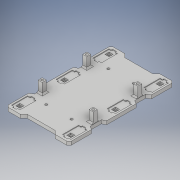
# Autodesk Inventor part: BODY_BOTTOM
Saved by Autodesk Inventor 2017.3 (Build 213256000, 256)
## iProperties
Created: 2017-08-24
Part Number: BODY_BOTTOM
Material: Generic
Document SubType Name: Modeling
Designer: Alexander Miller
Density: 1 g/cm^3
Appearance: Default
body_A: 150,000 mm
body_B: 90,000 mm
body_C: 5,000 mm
Author: Alexander Miller
Autodesk Inventor part; units mm, degrees
ref_plane "YZ Plane" through (0, 0, 0) normal (1, 0, 0) x (0, 1, 0)
ref_plane "XZ Plane" through (0, 0, 0) normal (0, 1, 0) x (-1, 0, 0)
ref_plane "XY Plane" through (0, 0, 0) normal (0, 0, 1) x (1, 0, 0)
sketch "Sketch4" plane through (0, 0, 0) normal (0, 1, 0) x (-1, 0, 0)
  line L0 (45, 75) -> (-45, 75)
  line L1 (-45, 75) -> (-45, -75)
  line L2 (-45, -75) -> (45, -75)
  line L3 (45, -75) -> (45, 75)
  point P0 (0, 0)
  point P1 (0, -75)
  point P2 (45, 0)
  dimension "d15" = 150
  dimension "d16" = 90
  constraints: 8 end point, 2 midpoint, 2 parallel, 1 horizontal, 1 horizontal alignment, 1 perpendicular, 1 vertical alignment
  measures "d15" distance of L2.end L0.start
  measures "d16" distance of L1.end L2.end
extrude "BodyPlate" add sketch "Sketch4" along normal blind 5
sketch "Sketch5" plane through (0, 5, 0) normal (0, 1, 0) x (1, 0, 0)
  line L0 (-42.5, 69.75) -> (-30.5, 69.75)
  line L1 (-30.5, 69.75) -> (-30.5, 46.75)
  line L2 (-30.5, 46.75) -> (-42.5, 46.75)
  line L3 (-42.5, 46.75) -> (-42.5, 69.75)
  line L4 (-42.5, 17) -> (-30.5, 17)
  line L5 (-30.5, 17) -> (-30.5, -6)
  line L6 (-30.5, -6) -> (-42.5, -6)
  line L7 (-42.5, -6) -> (-42.5, 17)
  line L8 (-42.5, -46.75) -> (-30.5, -46.75)
  line L9 (-30.5, -46.75) -> (-30.5, -69.75)
  line L10 (-30.5, -69.75) -> (-42.5, -69.75)
  line L11 (-42.5, -69.75) -> (-42.5, -46.75)
  line L12 (45, 75) -> (-45, 75) projected
  line L13 (-45, 75) -> (-45, -75) projected
  line L14 (-45, -75) -> (45, -75) projected
  circle A0 centre (-36.5, 0) radius 6 construction
  line L15 (0, 105) -> (0, -105) construction
  line L16 (42.5, 69.75) -> (30.5, 69.75)
  line L17 (30.5, 69.75) -> (30.5, 46.75)
  line L18 (30.5, 46.75) -> (42.5, 46.75)
  line L19 (42.5, 46.75) -> (42.5, 69.75)
  line L20 (42.5, 17) -> (30.5, 17)
  line L21 (30.5, 17) -> (30.5, -6)
  line L22 (30.5, -6) -> (42.5, -6)
  line L23 (42.5, -6) -> (42.5, 17)
  line L24 (42.5, -46.75) -> (30.5, -46.75)
  line L25 (30.5, -46.75) -> (30.5, -69.75)
  line L26 (30.5, -69.75) -> (42.5, -69.75)
  line L27 (42.5, -69.75) -> (42.5, -46.75)
  point P0 (0, 0)
  point P1 (-36.5, 46.75)
  point P2 (-36.5, 17)
  point P3 (-36.5, -6)
  point P4 (-36.5, -46.75)
  dimension "d19" = 23
  dimension "d20" = 12
  dimension "d21" = 5.25
  dimension "d22" = 2.5
  dimension "d23" = 5.25
  constraints: 48 end point, 12 symmetric about line, 6 parallel, 4 equal length, 4 midpoint, 3 horizontal, 3 perpendicular, 3 tangent, 2 vertical alignment, 1 centre point, 1 horizontal alignment
  measures "d19" distance of L2.end L0.start
  measures "d20" distance of L0.start L0.end
  measures "d21" distance between parallel lines of L0 L12
  measures "d22" distance between parallel lines of L3 L13
  measures "d23" distance between parallel lines of L14 L10
extrude "ServoIndentation" cut sketch "Sketch5" against normal blind 1
sketch "Sketch6" plane through (0, 5, 0) normal (0, 1, 0) x (1, 0, 0)
  line L0 (-39, 71.75) -> (-34, 71.75)
  line L1 (-34, 71.75) -> (-34, 69.75)
  line L2 (-34, 69.75) -> (-39, 69.75)
  line L3 (-39, 69.75) -> (-39, 71.75)
  line L4 (-39, 46.75) -> (-34, 46.75)
  line L5 (-34, 46.75) -> (-34, 44.75)
  line L6 (-34, 44.75) -> (-39, 44.75)
  line L7 (-39, 44.75) -> (-39, 46.75)
  line L8 (-42.5, 69.75) -> (-30.5, 69.75) projected
  line L9 (-30.5, 46.75) -> (-42.5, 46.75) projected
  line L10 (-39, 19) -> (-34, 19)
  line L11 (-34, 19) -> (-34, 17)
  line L12 (-34, 17) -> (-39, 17)
  line L13 (-39, 17) -> (-39, 19)
  line L14 (-39, -6) -> (-34, -6)
  line L15 (-34, -6) -> (-34, -8)
  line L16 (-34, -8) -> (-39, -8)
  line L17 (-39, -8) -> (-39, -6)
  line L18 (-39, -44.75) -> (-34, -44.75)
  line L19 (-34, -44.75) -> (-34, -46.75)
  line L20 (-34, -46.75) -> (-39, -46.75)
  line L21 (-39, -46.75) -> (-39, -44.75)
  line L22 (-39, -69.75) -> (-34, -69.75)
  line L23 (-34, -69.75) -> (-34, -71.75)
  line L24 (-34, -71.75) -> (-39, -71.75)
  line L25 (-39, -71.75) -> (-39, -69.75)
  line L26 (-42.5, 17) -> (-30.5, 17) projected
  line L27 (-30.5, -6) -> (-42.5, -6) projected
  line L28 (-42.5, -46.75) -> (-30.5, -46.75) projected
  line L29 (-30.5, -69.75) -> (-42.5, -69.75) projected
  line L30 (0, 105) -> (0, -105) projected
  line L31 (39, 71.75) -> (34, 71.75)
  line L32 (34, 71.75) -> (34, 69.75)
  line L33 (34, 69.75) -> (39, 69.75)
  line L34 (39, 69.75) -> (39, 71.75)
  line L35 (39, 46.75) -> (34, 46.75)
  line L36 (34, 46.75) -> (34, 44.75)
  line L37 (34, 44.75) -> (39, 44.75)
  line L38 (39, 44.75) -> (39, 46.75)
  line L39 (39, 19) -> (34, 19)
  line L40 (34, 19) -> (34, 17)
  line L41 (34, 17) -> (39, 17)
  line L42 (39, 17) -> (39, 19)
  line L43 (39, -6) -> (34, -6)
  line L44 (34, -6) -> (34, -8)
  line L45 (34, -8) -> (39, -8)
  line L46 (39, -8) -> (39, -6)
  line L47 (39, -44.75) -> (34, -44.75)
  line L48 (34, -44.75) -> (34, -46.75)
  line L49 (34, -46.75) -> (39, -46.75)
  line L50 (39, -46.75) -> (39, -44.75)
  line L51 (39, -69.75) -> (34, -69.75)
  line L52 (34, -69.75) -> (34, -71.75)
  line L53 (34, -71.75) -> (39, -71.75)
  line L54 (39, -71.75) -> (39, -69.75)
  point P0 (0, 0)
  point P1 (-36.5, 69.75)
  point P2 (-36.5, 69.75)
  point P3 (-36.5, 46.75)
  point P4 (-36.5, 46.75)
  point P5 (-36.5, 17)
  point P6 (-36.5, 17)
  point P7 (-36.5, -6)
  point P8 (-36.5, -6)
  point P9 (-36.5, -46.75)
  point P10 (-36.5, -46.75)
  point P11 (-36.5, -69.75)
  point P12 (-36.5, -69.75)
  dimension "d28" = 2
  dimension "d29" = 5
  constraints: 96 end point, 24 symmetric about line, 12 midpoint, 12 parallel, 9 equal length, 6 coincident, 6 collinear, 6 horizontal, 6 perpendicular, 2 point on line
  measures "d28" distance of L2.end L0.start
  measures "d29" distance of L0.start L0.end
extrude "ServoCableIdentation" cut sketch "Sketch6" against normal up to surface (1 mm away)
fillet "ServoCableFillet" radius 0.75 24 edges at (-39, 4.5, -69.75) (-34, 4.5, -69.75) (-39, 4.5, -46.75) (-34, 4.5, -46.75) (-39, 4.5, -17) (-34, 4.5, -17) (-39, 4.5, 6) (-34, 4.5, 6) (-39, 4.5, 46.75) (-34, 4.5, 46.75) (-39, 4.5, 69.75) (-34, 4.5, 69.75) (34, 4.5, -69.75) (39, 4.5, -69.75) (34, 4.5, -46.75) (39, 4.5, -46.75) (34, 4.5, -17) (39, 4.5, -17) (34, 4.5, 6) (39, 4.5, 6) (34, 4.5, 46.75) (39, 4.5, 46.75) (34, 4.5, 69.75) (39, 4.5, 69.75)
sketch "Sketch7" plane through (0, 5, 0) normal (0, 1, 0) x (1, 0, 0)
  line L0 (45, 75) -> (-45, 75) projected
  circle A0 centre (-18.1, 44.45) radius 1.675
  circle A1 centre (-18.1, -44.45) radius 1.675
  circle A2 centre (18.1, 44.45) radius 1.675
  circle A3 centre (18.1, -44.45) radius 1.675
  line L1 (-18.1, -44.45) -> (18.1, -44.45) construction
  line L2 (18.1, -44.45) -> (18.1, 44.45) construction
  line L3 (18.1, 44.45) -> (-18.1, 44.45) construction
  line L4 (-18.1, 44.45) -> (-18.1, -44.45) construction
  point P0 (0, 0)
  point P1 (-18.1, 0)
  point P2 (0, 44.45)
  dimension "d40" = 88.9
  dimension "d63" = 36.2
  dimension "d65" = 3.35
  constraints: 8 end point, 4 centre point, 3 equal radius, 3 horizontal alignment, 3 vertical alignment, 2 midpoint, 2 parallel, 1 horizontal, 1 perpendicular
  measures "d40" distance of A0.centre L1.start
  measures "d63" distance of A3.centre L1.start
  measures "d65" diameter of A0
extrude "PCBMounting" cut sketch "Sketch7" against normal through all
sketch "Sketch8" plane through (0, 0, 0) normal (0, -1, 0) x (1, 0, 0)
  circle A0 centre (18.1, -44.45) radius 1.675 projected
  circle A1 centre (-18.1, -44.45) radius 1.675 projected
  circle A2 centre (-18.1, 44.45) radius 1.675 projected
  circle A3 centre (18.1, 44.45) radius 1.675 projected
  line L0 (15.175, 47.375) -> (21.025, 47.375)
  line L1 (21.025, 47.375) -> (21.025, 41.525)
  line L2 (21.025, 41.525) -> (15.175, 41.525)
  line L3 (15.175, 41.525) -> (15.175, 47.375)
  line L4 (15.175, -41.525) -> (21.025, -41.525)
  line L5 (21.025, -41.525) -> (21.025, -47.375)
  line L6 (21.025, -47.375) -> (15.175, -47.375)
  line L7 (15.175, -47.375) -> (15.175, -41.525)
  line L8 (-21.025, -41.525) -> (-15.175, -41.525)
  line L9 (-15.175, -41.525) -> (-15.175, -47.375)
  line L10 (-15.175, -47.375) -> (-21.025, -47.375)
  line L11 (-21.025, -47.375) -> (-21.025, -41.525)
  line L12 (-21.025, 47.375) -> (-15.175, 47.375)
  line L13 (-15.175, 47.375) -> (-15.175, 41.525)
  line L14 (-15.175, 41.525) -> (-21.025, 41.525)
  line L15 (-21.025, 41.525) -> (-21.025, 47.375)
  point P0 (0, 0)
  point P1 (15.175, 44.45)
  point P2 (-15.175, 44.45)
  point P3 (-15.175, -44.45)
  point P4 (15.175, -44.45)
  point P5 (18.1, 41.525)
  point P6 (18.1, -41.525)
  point P7 (-18.1, -41.525)
  point P8 (-18.1, 41.525)
  dimension "d64" = 5.85
  constraints: 32 end point, 8 midpoint, 8 parallel, 6 equal length, 4 horizontal, 4 horizontal alignment, 4 perpendicular, 4 vertical alignment, 1 point on line
  measures "d64" distance of L1.end L2.end
extrude "PCBNuts" cut sketch "Sketch8" against normal blind 2.15
sketch "Sketch9" plane through (0, 5, 0) normal (0, 1, 0) x (1, 0, 0)
  line L0 (45, 42.875) -> (45, 20.875)
  line L1 (45, 20.875) -> (40, 23.875)
  line L2 (40, 23.875) -> (40, 39.875)
  line L3 (40, 39.875) -> (45, 42.875)
  line L4 (34, 44.75) -> (39, 44.75) projected
  line L5 (36.5, 44.75) -> (36.5, 19) construction
  line L6 (39, 19) -> (34, 19) projected
  line L7 (45, -75) -> (45, 75) projected
  line L8 (-63, 0) -> (63, 0) projected
  line L9 (0, 105) -> (0, -105) projected
  line L10 (-45, 42.875) -> (-45, 20.875)
  line L11 (-45, 20.875) -> (-40, 23.875)
  line L12 (-40, 23.875) -> (-40, 39.875)
  line L13 (-40, 39.875) -> (-45, 42.875)
  line L14 (25, 75) -> (-25, 75)
  line L15 (-25, 75) -> (-20, 70)
  line L16 (-20, 70) -> (20, 70)
  line L17 (20, 70) -> (25, 75)
  line L18 (45, 75) -> (-45, 75) projected
  line L19 (45, -42.875) -> (45, -20.875)
  line L20 (45, -20.875) -> (40, -23.875)
  line L21 (40, -23.875) -> (40, -39.875)
  line L22 (40, -39.875) -> (45, -42.875)
  line L23 (-40, -39.875) -> (-45, -42.875)
  line L24 (-45, -42.875) -> (-45, -20.875)
  line L25 (-45, -20.875) -> (-40, -23.875)
  line L26 (-40, -23.875) -> (-40, -39.875)
  line L27 (25, -75) -> (-25, -75)
  line L28 (-25, -75) -> (-20, -70)
  line L29 (-20, -70) -> (20, -70)
  line L30 (20, -70) -> (25, -75)
  point P0 (0, 0)
  point P1 (45, 31.875)
  point P2 (40, 31.875)
  point P3 (36.5, 31.875)
  point P4 (0, 75)
  point P5 (0, 70)
  dimension "d46" = 5
  dimension "d47" = 16
  dimension "d48" = 22
  dimension "d49" = 5
  dimension "d50" = 40
  dimension "d51" = 50
  constraints: 50 end point, 16 symmetric about line, 7 midpoint, 2 collinear, 2 horizontal alignment, 2 parallel, 2 vertical alignment, 1 horizontal, 1 vertical
  measures "d46" distance between parallel lines of L2 L0
  measures "d47" distance of L1.end L2.end
  measures "d48" distance of L0.start L0.end
  measures "d49" distance between parallel lines of L16 L14
  measures "d50" distance of L15.end L16.end
  measures "d51" distance of L14.start L14.end
extrude "BodyIndentation" cut sketch "Sketch9" against normal through all contours L0 L1 L2 L3 | L17 L16 L9 L14 | L9 L16 L15 L14 | L22 L21 L20 L7 | L29 L30 L27 L9 | L9 L27 L28 L29 | L13 L12 L11 L10 | L23 L24 L25 L26
chamfer "BodyChamfer" distance 3 angle 45 4 edges at (-45, 2.5, 75) (-45, 2.5, -75) (45, 2.5, 75) (45, 2.5, -75)
sketch "Sketch10" plane through (0, 4, 0) normal (0, 1, 0) x (1, 0, 0)
  line L0 (-39.425, 66.675) -> (-33.575, 66.675)
  line L1 (-33.575, 66.675) -> (-33.575, 60.825)
  line L2 (-33.575, 60.825) -> (-39.425, 60.825)
  line L3 (-39.425, 60.825) -> (-39.425, 66.675)
  line L4 (-39.425, -2.925) -> (-33.575, -2.925)
  line L5 (-33.575, -2.925) -> (-33.575, 2.925)
  line L6 (-33.575, 2.925) -> (-39.425, 2.925)
  line L7 (-39.425, 2.925) -> (-39.425, -2.925)
  line L8 (-39.425, -66.675) -> (-33.575, -66.675)
  line L9 (-33.575, -66.675) -> (-33.575, -60.825)
  line L10 (-33.575, -60.825) -> (-39.425, -60.825)
  line L11 (-39.425, -60.825) -> (-39.425, -66.675)
  line L12 (-42.5, 46.75) -> (-42.5, 69.75) construction
  line L13 (-33.25, 69.75) -> (-30.5, 69.75) construction
  line L14 (-42.5, 69.75) -> (-30.5, 69.75) construction
  circle A0 centre (-36.5, 63.75) radius 6 construction
  line L15 (-30.5, 69.75) -> (-30.5, 46.75) construction
  line L16 (-39.75, -6) -> (-42.5, -6) construction
  line L17 (-42.5, -6) -> (-30.5, -6) construction
  circle A1 centre (-36.5, 0) radius 6 construction
  line L18 (-42.5, -6) -> (-42.5, 17) construction
  line L19 (-30.5, 17) -> (-30.5, -6) construction
  line L20 (-30.5, -46.75) -> (-30.5, -69.75) construction
  line L21 (-42.5, -69.75) -> (-42.5, -46.75) construction
  line L22 (-30.5, -69.75) -> (-42.5, -69.75) construction
  circle A2 centre (-36.5, -63.75) radius 6 construction
  line L23 (0, 105) -> (0, -105) construction
  line L24 (39.425, 66.675) -> (33.575, 66.675)
  line L25 (33.575, 66.675) -> (33.575, 60.825)
  line L26 (33.575, 60.825) -> (39.425, 60.825)
  line L27 (39.425, 60.825) -> (39.425, 66.675)
  line L28 (39.425, -2.925) -> (33.575, -2.925)
  line L29 (33.575, -2.925) -> (33.575, 2.925)
  line L30 (33.575, 2.925) -> (39.425, 2.925)
  line L31 (39.425, 2.925) -> (39.425, -2.925)
  line L32 (39.425, -66.675) -> (33.575, -66.675)
  line L33 (33.575, -66.675) -> (33.575, -60.825)
  line L34 (33.575, -60.825) -> (39.425, -60.825)
  line L35 (39.425, -60.825) -> (39.425, -66.675)
  point P0 (0, 0)
  point P1 (-36.5, 60.825)
  point P2 (-36.5, 2.925)
  point P3 (-36.5, -2.925)
  point P4 (-36.5, -60.825)
  point P5 (-36.5, 69.75)
  point P6 (-39.425, 63.75)
  point P7 (-36.5, 66.675)
  point P8 (-33.575, 0)
  point P9 (-33.575, -63.75)
  point P10 (36.5, 60.825)
  point P11 (36.5, 2.925)
  point P12 (36.5, -2.925)
  point P13 (36.5, -60.825)
  point P14 (36.5, 63.75)
  point P15 (39.425, 63.75)
  point P16 (36.5, 66.675)
  point P17 (36.5, 0)
  point P18 (33.575, 0)
  point P19 (36.5, -63.75)
  point P20 (33.575, -63.75)
  dimension "d57" = 5.85
  constraints: 54 end point, 23 symmetric about line, 9 midpoint, 8 perpendicular, 8 tangent, 6 parallel, 4 horizontal, 4 vertical alignment, 3 centre point, 3 horizontal alignment, 2 collinear
  measures "d57" distance of L0.end L1.end
extrude "BallbearingNut" cut sketch "Sketch10" against normal blind 2.15
sketch "Sketch11" plane through (0, 1.85, 0) normal (0, 1, 0) x (1, 0, 0)
  circle A0 centre (-36.5, -63.75) radius 1.675
  circle A1 centre (-36.5, 0) radius 1.675
  circle A2 centre (-36.5, 63.75) radius 1.675
  line L0 (0, 105) -> (0, -105) projected
  line L1 (-39.425, -66.675) -> (-39.425, -60.825) projected
  line L2 (-33.575, -66.675) -> (-39.425, -66.675) projected
  line L3 (-39.425, -2.925) -> (-39.425, 2.925) projected
  line L4 (-39.425, 60.825) -> (-39.425, 66.675) projected
  circle A3 centre (36.5, -63.75) radius 1.675
  circle A4 centre (36.5, 0) radius 1.675
  circle A5 centre (36.5, 63.75) radius 1.675
  point P0 (0, 0)
  point P1 (-39.425, -63.75)
  point P2 (-36.5, -66.675)
  point P3 (-39.425, 0)
  point P4 (-39.425, 63.75)
  dimension "d60" = 3.35
  constraints: 6 centre point, 4 midpoint, 3 horizontal alignment, 3 symmetric about line, 3 vertical alignment, 2 equal radius, 3 other
  measures "d60" diameter of A0
extrude "BallbearingMounting" cut sketch "Sketch11" against normal through all
sketch "Sketch12" plane through (0, 5, 0) normal (0, 1, 0) x (1, 0, 0)
  circle A0 centre (-36.5, -31.875) radius 1.675
  line L0 (-40, -23.875) -> (-40, -39.875) projected
  line L1 (-39, -44.75) -> (-34, -44.75) projected
  line L2 (-63, 0) -> (63, 0) projected
  line L3 (0, 105) -> (0, -105) projected
  circle A1 centre (-36.5, 31.875) radius 1.675
  circle A2 centre (36.5, -31.875) radius 1.675
  circle A3 centre (36.5, 31.875) radius 1.675
  point P0 (0, 0)
  point P1 (-40, -31.875)
  point P2 (-36.5, -44.75)
  dimension "d66" = 3.35
  constraints: 4 centre point, 3 symmetric about line, 2 midpoint, 1 horizontal alignment, 1 vertical alignment, 3 other
  measures "d66" diameter of A0
extrude "PlateMounting" cut sketch "Sketch12" against normal through all
sketch "Sketch13" plane through (0, 0, 0) normal (0, -1, 0) x (1, 0, 0)
  line L0 (33.575, 34.8) -> (39.425, 34.8)
  line L1 (39.425, 34.8) -> (39.425, 28.95)
  line L2 (39.425, 28.95) -> (33.575, 28.95)
  line L3 (33.575, 28.95) -> (33.575, 34.8)
  circle A0 centre (36.5, 31.875) radius 1.675 projected
  line L4 (-63, 0) -> (63, 0) projected
  line L5 (0, -105) -> (0, 105) projected
  line L6 (33.575, -34.8) -> (39.425, -34.8)
  line L7 (39.425, -34.8) -> (39.425, -28.95)
  line L8 (39.425, -28.95) -> (33.575, -28.95)
  line L9 (33.575, -28.95) -> (33.575, -34.8)
  line L10 (-33.575, 34.8) -> (-39.425, 34.8)
  line L11 (-39.425, 34.8) -> (-39.425, 28.95)
  line L12 (-39.425, 28.95) -> (-33.575, 28.95)
  line L13 (-33.575, 28.95) -> (-33.575, 34.8)
  line L14 (-33.575, -34.8) -> (-39.425, -34.8)
  line L15 (-39.425, -34.8) -> (-39.425, -28.95)
  line L16 (-39.425, -28.95) -> (-33.575, -28.95)
  line L17 (-33.575, -28.95) -> (-33.575, -34.8)
  point P0 (0, 0)
  point P1 (36.5, 28.95)
  point P2 (39.425, 31.875)
  dimension "d69" = 5.85
  constraints: 32 end point, 12 symmetric about line, 2 midpoint, 2 parallel, 2 perpendicular, 1 horizontal, 1 horizontal alignment, 1 vertical alignment
  measures "d69" distance of L1.end L2.end
extrude "PlateNuts" cut sketch "Sketch13" against normal blind 2.15
sketch "Sketch14" plane through (0, 5, 0) normal (0, 1, 0) x (1, 0, 0)
  circle A0 centre (36.5, -31.875) radius 1.675 projected
  circle A1 centre (-36.5, -31.875) radius 1.675 projected
  circle A2 centre (-36.5, 31.875) radius 1.675 projected
  circle A3 centre (36.5, 31.875) radius 1.675 projected
  line L0 (42, 75) -> (45, 72) projected
  line L1 (42, 75) -> (25, 75) projected
  line L2 (25, 75) -> (20, 70) projected
  line L3 (20, 70) -> (-20, 70) projected
  line L4 (-20, 70) -> (-25, 75) projected
  line L5 (-25, 75) -> (-42, 75) projected
  line L6 (-45, 72) -> (-42, 75) projected
  line L7 (-45, 72) -> (-45, 42.875) projected
  line L8 (-45, 42.875) -> (-40, 39.875) projected
  line L9 (-40, 39.875) -> (-40, 23.875) projected
  line L10 (-40, 23.875) -> (-45, 20.875) projected
  line L11 (-45, 20.875) -> (-45, -20.875) projected
  line L12 (-45, -20.875) -> (-40, -23.875) projected
  line L13 (-40, -23.875) -> (-40, -39.875) projected
  line L14 (-40, -39.875) -> (-45, -42.875) projected
  line L15 (-45, -42.875) -> (-45, -72) projected
  line L16 (-42, -75) -> (-45, -72) projected
  line L17 (-42, -75) -> (-25, -75) projected
  line L18 (-25, -75) -> (-20, -70) projected
  line L19 (-20, -70) -> (20, -70) projected
  line L20 (20, -70) -> (25, -75) projected
  line L21 (25, -75) -> (42, -75) projected
  line L22 (45, -72) -> (42, -75) projected
  line L23 (45, -72) -> (45, -42.875) projected
  line L24 (45, -42.875) -> (40, -39.875) projected
  line L25 (40, -39.875) -> (40, -23.875) projected
  line L26 (40, -23.875) -> (45, -20.875) projected
  line L27 (45, -20.875) -> (45, 20.875) projected
  line L28 (45, 20.875) -> (40, 23.875) projected
  line L29 (40, 23.875) -> (40, 39.875) projected
  line L30 (40, 39.875) -> (45, 42.875) projected
  line L31 (45, 42.875) -> (45, 72) projected
  arc A4 (-33.25, 46.75) -> (-34, 46) centre (-33.25, 46) ccw projected
  line L32 (-34, 46) -> (-34, 44.75) projected
  line L33 (-34, 44.75) -> (-39, 44.75) projected
  line L34 (-39, 44.75) -> (-39, 46) projected
  arc A5 (-39, 46) -> (-39.75, 46.75) centre (-39.75, 46) ccw projected
  line L35 (-39.75, 46.75) -> (-42.5, 46.75) projected
  line L36 (-42.5, 46.75) -> (-42.5, 69.75) projected
  line L37 (-42.5, 69.75) -> (-39.75, 69.75) projected
  arc A6 (-39.75, 69.75) -> (-39, 70.5) centre (-39.75, 70.5) ccw projected
  line L38 (-39, 70.5) -> (-39, 71.75) projected
  line L39 (-39, 71.75) -> (-34, 71.75) projected
  line L40 (-34, 71.75) -> (-34, 70.5) projected
  arc A7 (-34, 70.5) -> (-33.25, 69.75) centre (-33.25, 70.5) ccw projected
  line L41 (-33.25, 69.75) -> (-30.5, 69.75) projected
  line L42 (-30.5, 69.75) -> (-30.5, 46.75) projected
  line L43 (-30.5, 46.75) -> (-33.25, 46.75) projected
  arc A8 (-33.25, -6) -> (-34, -6.75) centre (-33.25, -6.75) ccw projected
  line L44 (-34, -6.75) -> (-34, -8) projected
  line L45 (-34, -8) -> (-39, -8) projected
  line L46 (-39, -8) -> (-39, -6.75) projected
  arc A9 (-39, -6.75) -> (-39.75, -6) centre (-39.75, -6.75) ccw projected
  line L47 (-39.75, -6) -> (-42.5, -6) projected
  line L48 (-42.5, -6) -> (-42.5, 17) projected
  line L49 (-42.5, 17) -> (-39.75, 17) projected
  arc A10 (-39.75, 17) -> (-39, 17.75) centre (-39.75, 17.75) ccw projected
  line L50 (-39, 17.75) -> (-39, 19) projected
  line L51 (-39, 19) -> (-34, 19) projected
  line L52 (-34, 19) -> (-34, 17.75) projected
  arc A11 (-34, 17.75) -> (-33.25, 17) centre (-33.25, 17.75) ccw projected
  line L53 (-33.25, 17) -> (-30.5, 17) projected
  line L54 (-30.5, 17) -> (-30.5, -6) projected
  line L55 (-30.5, -6) -> (-33.25, -6) projected
  arc A12 (-33.25, -69.75) -> (-34, -70.5) centre (-33.25, -70.5) ccw projected
  line L56 (-34, -70.5) -> (-34, -71.75) projected
  line L57 (-34, -71.75) -> (-39, -71.75) projected
  line L58 (-39, -71.75) -> (-39, -70.5) projected
  arc A13 (-39, -70.5) -> (-39.75, -69.75) centre (-39.75, -70.5) ccw projected
  line L59 (-39.75, -69.75) -> (-42.5, -69.75) projected
  line L60 (-42.5, -69.75) -> (-42.5, -46.75) projected
  line L61 (-42.5, -46.75) -> (-39.75, -46.75) projected
  arc A14 (-39.75, -46.75) -> (-39, -46) centre (-39.75, -46) ccw projected
  line L62 (-39, -46) -> (-39, -44.75) projected
  line L63 (-39, -44.75) -> (-34, -44.75) projected
  line L64 (-34, -44.75) -> (-34, -46) projected
  arc A15 (-34, -46) -> (-33.25, -46.75) centre (-33.25, -46) ccw projected
  line L65 (-33.25, -46.75) -> (-30.5, -46.75) projected
  line L66 (-30.5, -46.75) -> (-30.5, -69.75) projected
  line L67 (-30.5, -69.75) -> (-33.25, -69.75) projected
  arc A16 (39.75, 46.75) -> (39, 46) centre (39.75, 46) ccw projected
  line L68 (39, 46) -> (39, 44.75) projected
  line L69 (39, 44.75) -> (34, 44.75) projected
  line L70 (34, 44.75) -> (34, 46) projected
  arc A17 (34, 46) -> (33.25, 46.75) centre (33.25, 46) ccw projected
  line L71 (33.25, 46.75) -> (30.5, 46.75) projected
  line L72 (30.5, 46.75) -> (30.5, 69.75) projected
  line L73 (30.5, 69.75) -> (33.25, 69.75) projected
  arc A18 (33.25, 69.75) -> (34, 70.5) centre (33.25, 70.5) ccw projected
  line L74 (34, 70.5) -> (34, 71.75) projected
  line L75 (34, 71.75) -> (39, 71.75) projected
  line L76 (39, 71.75) -> (39, 70.5) projected
  arc A19 (39, 70.5) -> (39.75, 69.75) centre (39.75, 70.5) ccw projected
  line L77 (39.75, 69.75) -> (42.5, 69.75) projected
  line L78 (42.5, 69.75) -> (42.5, 46.75) projected
  line L79 (42.5, 46.75) -> (39.75, 46.75) projected
  arc A20 (39.75, -6) -> (39, -6.75) centre (39.75, -6.75) ccw projected
  line L80 (39, -6.75) -> (39, -8) projected
  line L81 (39, -8) -> (34, -8) projected
  line L82 (34, -8) -> (34, -6.75) projected
  arc A21 (34, -6.75) -> (33.25, -6) centre (33.25, -6.75) ccw projected
  line L83 (33.25, -6) -> (30.5, -6) projected
  line L84 (30.5, -6) -> (30.5, 17) projected
  line L85 (30.5, 17) -> (33.25, 17) projected
  arc A22 (33.25, 17) -> (34, 17.75) centre (33.25, 17.75) ccw projected
  line L86 (34, 17.75) -> (34, 19) projected
  line L87 (34, 19) -> (39, 19) projected
  line L88 (39, 19) -> (39, 17.75) projected
  arc A23 (39, 17.75) -> (39.75, 17) centre (39.75, 17.75) ccw projected
  line L89 (39.75, 17) -> (42.5, 17) projected
  line L90 (42.5, 17) -> (42.5, -6) projected
  line L91 (42.5, -6) -> (39.75, -6) projected
  arc A24 (39.75, -69.75) -> (39, -70.5) centre (39.75, -70.5) ccw projected
  line L92 (39, -70.5) -> (39, -71.75) projected
  line L93 (39, -71.75) -> (34, -71.75) projected
  line L94 (34, -71.75) -> (34, -70.5) projected
  arc A25 (34, -70.5) -> (33.25, -69.75) centre (33.25, -70.5) ccw projected
  line L95 (33.25, -69.75) -> (30.5, -69.75) projected
  line L96 (30.5, -69.75) -> (30.5, -46.75) projected
  line L97 (30.5, -46.75) -> (33.25, -46.75) projected
  arc A26 (33.25, -46.75) -> (34, -46) centre (33.25, -46) ccw projected
  line L98 (34, -46) -> (34, -44.75) projected
  line L99 (34, -44.75) -> (39, -44.75) projected
  line L100 (39, -44.75) -> (39, -46) projected
  arc A27 (39, -46) -> (39.75, -46.75) centre (39.75, -46) ccw projected
  line L101 (39.75, -46.75) -> (42.5, -46.75) projected
  line L102 (42.5, -46.75) -> (42.5, -69.75) projected
  line L103 (42.5, -69.75) -> (39.75, -69.75) projected
  circle A28 centre (18.1, -44.45) radius 1.675 projected
  circle A29 centre (-18.1, -44.45) radius 1.675 projected
  circle A30 centre (-18.1, 44.45) radius 1.675 projected
  circle A31 centre (18.1, 44.45) radius 1.675 projected
  line L104 (-33.575, 28.95) -> (-33.575, 34.8) projected
  line L105 (-39.425, 28.95) -> (-33.575, 28.95) projected
  line L106 (-39.425, 34.8) -> (-39.425, 28.95) projected
  line L107 (-33.575, 34.8) -> (-39.425, 34.8) projected
  line L108 (39.425, -34.8) -> (39.425, -28.95) projected
  line L109 (39.425, -28.95) -> (33.575, -28.95) projected
  line L110 (33.575, -28.95) -> (33.575, -34.8) projected
  line L111 (33.575, -34.8) -> (39.425, -34.8) projected
  line L112 (33.575, 34.8) -> (33.575, 28.95) projected
  line L113 (33.575, 28.95) -> (39.425, 28.95) projected
  line L114 (39.425, 28.95) -> (39.425, 34.8) projected
  line L115 (39.425, 34.8) -> (33.575, 34.8) projected
  line L116 (-21.025, -41.525) -> (-21.025, -47.375) projected
  line L117 (-39.425, -34.8) -> (-33.575, -34.8) projected
  line L118 (-33.575, -34.8) -> (-33.575, -28.95) projected
  line L119 (-33.575, -28.95) -> (-39.425, -28.95) projected
  line L120 (-39.425, -28.95) -> (-39.425, -34.8) projected
  point P0 (0, 0)
extrude "Extrusion13" add sketch "Sketch14" along normal blind 15 contours L105 L106 L107 L104 | L111 L110 L109 L108 | L115 L114 L113 L112 | L120 L119 L118 L117
chamfer "Chamfer2" distance 2 angle 45 12 edges at (36.5, 5, 28.95) (36.5, 5, 34.8) (33.575, 5, 31.875) (36.5, 5, -28.95) (33.575, 5, -31.875) (36.5, 5, -34.8) (-36.5, 5, -34.8) (-33.575, 5, -31.875) (-36.5, 5, -28.95) (-36.5, 5, 28.95) (-33.575, 5, 31.875) (-36.5, 5, 34.8)
equation "\"d15\" = body_A"
equation "\"d16\" = body_B"
equation "\"d17\" = body_C"
equation "\"d19\" = servo_A"
equation "\"d20\" = servo_B"
equation "\"d22\" = 0.5 * body_C"
equation "\"d23\" = d21"
equation "\"body_A\" = 150"
equation "\"body_B\" = 90"
equation "\"body_C\" = 5"
equation "\"body_D\" = 0.25 * servo_D"
equation "\"body_E\" = 0.25 * servo_D"
equation "\"servo_A\" = 23"
equation "\"servo_B\" = 12"
equation "\"servo_D\" = 31.5"
body "Solid2"
